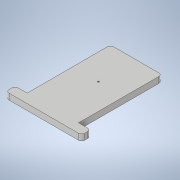
# Autodesk Inventor part: 00_Slider_Mask_Darkfield
Saved by Autodesk Inventor 2022.3 (Build 263350000, 350)
## iProperties
Created: 2021-10-22
Part Number: 00_Slider_Mask_Darkfield
Material: Generic
Document SubType Name: Modeling
Designer: diederichbenedict
Density: 1 g/cm^3
Appearance: Default
Author: diederichbenedict
Autodesk Inventor part; units mm, degrees
ref_plane "YZ Plane" through (0, 0, 0) normal (1, 0, 0) x (0, 1, 0)
ref_plane "XZ Plane" through (0, 0, 0) normal (0, 1, 0) x (-1, 0, 0)
ref_plane "XY Plane" through (0, 0, 0) normal (0, 0, 1) x (1, 0, 0)
sketch "Sketch1" plane through (0, 0, 0) normal (0, 1, 0) x (-1, 0, 0)
  line L0 (-17, 30.1) -> (17, 30.1)
  line L1 (17, 30.1) -> (17, 25)
  line L2 (17, -25) -> (-17, -25)
  line L3 (-17, -25) -> (-17, 25)
  line L4 (9, -19.575) -> (9, 19.575)
  line L5 (9, 19.575) -> (-9, 19.575)
  line L6 (-9, 19.575) -> (-9, -19.575)
  line L7 (-9, -19.575) -> (9, -19.575)
  line L8 (-25, 36.1) -> (25, 36.1)
  line L9 (25, 36.1) -> (25, 30.1)
  line L10 (25, 30.1) -> (-25, 30.1)
  line L11 (-25, 30.1) -> (-25, 36.1)
  line L12 (-25, 36.1) -> (25, 30.1) construction
  line L13 (25, 36.1) -> (-25, 30.1) construction
  line L14 (17, 25) -> (-17, 25)
  line L15 (-17, 25) -> (-17, 30.1)
  line L16 (17, 25) -> (17, -25)
  point P0 (0, 0)
  point P1 (0, 33.1)
  point P2 (0, 30.1)
  point P3 (0, 0)
  point P4 (-17, 0)
  point P5 (-9, 0)
  dimension "d0" = 34
  dimension "d1" = 55.1
  dimension "d2" = 8
  dimension "d3" = 50
  dimension "d4" = 6
  dimension "d18" = 5.1
  dimension "d19" = 50
  dimension "d20" = 25
  constraints: 34 end point, 9 parallel, 6 midpoint, 6 perpendicular, 2 horizontal, 2 horizontal alignment
  measures "d0" distance of L2.start L2.end
  measures "d1" distance of L0.end L2.start
  measures "d2" distance between parallel lines of L1 L4
  measures "d3" distance of L9.end L10.end
  measures "d4" distance of L8.end L9.end
  measures "d18" distance between parallel lines of L14 L0
  measures "d19" distance between parallel lines of L2 L14
  measures "d20" distance from line of L14 point (0, 0)
extrude "Extrusion1" add sketch "Sketch1" along normal blind 4 contours L10 L11 L8 L9 L0 | L0 L1 L14 L15 | L14 L16 L2 L3 | L7 L6 L5 L4
sketch "Sketch2" plane through (0, 4, 0) normal (0, 1, 0) x (1, 0, 0)
  line L0 (25, -30.1) -> (17, -30.1) projected
  line L1 (-25, -30.1) -> (-25, -36.1) projected
  line L2 (-25, -36.1) -> (25, -36.1) projected
  line L3 (25, -36.1) -> (25, -30.1) projected
  line L4 (13.5, 17) -> (-13.5, 17)
  line L5 (-13.5, 17) -> (-13.5, -17)
  line L6 (-13.5, -17) -> (13.5, -17)
  line L7 (13.5, -17) -> (13.5, 17)
  line L8 (13.5, 17) -> (-13.5, -17) construction
  line L9 (-13.5, 17) -> (13.5, -17) construction
  circle A0 centre (0, 0) radius 13.5 construction
  circle A1 centre (0, 0) radius 0.5
  line L10 (-0.4, 0.3) -> (-13.9997, 0.3) construction
  line L11 (-13.9997, 0.3) -> (-13.9997, -0.3) construction
  line L12 (-13.9997, -0.3) -> (-0.4, -0.3) construction
  line L13 (-0.4, -0.3) -> (-0.4, 0.3) construction
  line L14 (0.4, 0.3) -> (13.9718, 0.3) construction
  line L15 (13.9718, 0.3) -> (13.9718, -0.3) construction
  line L16 (13.9718, -0.3) -> (0.4, -0.3) construction
  line L17 (0.4, -0.3) -> (0.4, 0.3) construction
  line L18 (17, -30.1) -> (17, 25) projected
  line L19 (17, 25) -> (-17, 25) projected
  line L20 (-17, 25) -> (-17, -30.1) projected
  line L21 (-17, -30.1) -> (-25, -30.1) projected
  point P0 (13.4967, -0.3)
  point P1 (13.5, -0.3)
  point P2 (13.5, 0)
  point P3 (13.5, 0.3)
  point P4 (13.4967, 0.3)
  point P5 (0.4, -0.3)
  point P6 (0.4, -0.3)
  point P7 (-0.4, -0.3)
  point P8 (-0.4, -0.3)
  point P9 (-13.4967, -0.3)
  point P10 (-13.5, -0.3)
  point P11 (-13.5, 0)
  point P12 (-13.4967, 0.3)
  point P13 (-13.5, 0.3)
  point P14 (-17, 0)
  dimension "d7" = 27
  dimension "d8" = 34
  dimension "d14" = 0.3
  dimension "d15" = 0.3
  dimension "d16" = 1
  constraints: 28 end point, 6 parallel, 3 horizontal, 3 midpoint, 3 perpendicular, 2 centre point, 2 coincident, 2 point on circle, 2 point on line, 1 horizontal alignment
  measures "d7" distance of L6.end L5.end
  measures "d8" distance of L5.end L4.end
  measures "d14" distance from line of point (0, 0) L10
  measures "d15" distance from line of point (0, 0) L12
  measures "d16" diameter of A1
extrude "Extrusion2" cut sketch "Sketch2" against normal through all draft 45 contours A1
sketch "Sketch3" plane through (0, 4, 0) normal (0, 1, 0) x (1, 0, 0)
  line L0 (-13.1847, -19.2539) -> (12.0411, -19.2539) construction
  line L1 (12.0411, -19.2539) -> (12.0411, -24.441) construction
  line L2 (12.0411, -24.441) -> (-13.1847, -24.441) construction
  line L3 (-13.1847, -24.441) -> (-13.1847, -19.2539) construction
  point P0 (0, 0)
  constraints: 2 other
extrude "Extrusion3" [suppressed]
fillet "Fillet1" radius 2 6 edges at (25, 2, 36.1) (25, 2, 30.1) (-25, 2, 36.1) (-25, 2, 30.1) (-17, 2, -25) (17, 2, -25)
sketch "Sketch4" plane through (0, 0, 0) normal (0, -1, 0) x (1, 0, 0)
  line L0 (-15.3446, -7.6834) -> (10.8174, -7.6834) construction
  line L1 (10.8174, -7.6834) -> (10.8174, -21.8309) construction
  line L2 (10.8174, -21.8309) -> (-15.3446, -21.8309) construction
  line L3 (-15.3446, -21.8309) -> (-15.3446, -7.6834) construction
  line L4 (-6.685, -13.4285) -> (-8.6364, -13.4285)
  line L5 (-8.6364, -13.4285) -> (-8.6364, -13.0201)
  line L6 (-8.6364, -13.0201) -> (-7.9103, -13.0201)
  line L7 (-7.9103, -13.0201) -> (-7.9103, -10.3394)
  line L8 (-7.9103, -10.3394) -> (-8.6364, -10.3394)
  line L9 (-8.6364, -10.3394) -> (-8.6364, -9.9731)
  spline S0 degree 2 poles (-8.6364, -9.9731) (-8.2247, -9.9731) (-7.8357, -9.7397) (-7.8098, -9.4156) knots 0 0 0 1 2 2 2
  line L10 (-7.8098, -9.4156) -> (-7.3949, -9.4156)
  line L11 (-7.3949, -9.4156) -> (-7.3949, -13.0201)
  line L12 (-7.3949, -13.0201) -> (-6.685, -13.0201)
  line L13 (-6.685, -13.0201) -> (-6.685, -13.4285)
  line L14 (-0.7531, -13.4285) -> (-0.7531, -11.6911)
  spline S1 degree 2 poles (-0.7531, -11.6911) (-0.7531, -11.4836) (-0.7855, -11.1303) (-0.8373, -11.0331) knots 0 0 0 1 2 2 2
  spline S2 degree 2 poles (-0.8373, -11.0331) (-0.8892, -10.9261) (-1.0869, -10.8224) (-1.2587, -10.8224) knots 0 0 0 1 2 2 2
  spline S3 degree 2 poles (-1.2587, -10.8224) (-1.4143, -10.8224) (-1.7709, -11.0136) (-1.9589, -11.1951) knots 0 0 0 1 2 2 2
  spline S4 degree 2 poles (-1.9589, -11.1951) (-1.9557, -11.2405) (-1.9492, -11.3669) (-1.9492, -11.4512) knots 0 0 0 1 2 2 2
  line L15 (-1.9492, -11.4512) -> (-1.9492, -13.4285)
  line L16 (-1.9492, -13.4285) -> (-2.4549, -13.4285)
  line L17 (-2.4549, -13.4285) -> (-2.4549, -11.6911)
  spline S5 degree 2 poles (-2.4549, -11.6911) (-2.4549, -11.4836) (-2.4873, -11.1303) (-2.5391, -11.0331) knots 0 0 0 1 2 2 2
  spline S6 degree 2 poles (-2.5391, -11.0331) (-2.591, -10.9261) (-2.7887, -10.8224) (-2.9605, -10.8224) knots 0 0 0 1 2 2 2
  spline S7 degree 2 poles (-2.9605, -10.8224) (-3.1226, -10.8224) (-3.4824, -11.0266) (-3.651, -11.1854) knots 0 0 0 1 2 2 2
  line L18 (-3.651, -11.1854) -> (-3.651, -13.4285)
  line L19 (-3.651, -13.4285) -> (-4.1566, -13.4285)
  line L20 (-4.1566, -13.4285) -> (-4.1566, -10.4269)
  line L21 (-4.1566, -10.4269) -> (-3.651, -10.4269)
  line L22 (-3.651, -10.4269) -> (-3.651, -10.7575)
  spline S8 degree 2 poles (-3.651, -10.7575) (-3.4532, -10.5598) (-3.0643, -10.3426) (-2.8309, -10.3426) knots 0 0 0 1 2 2 2
  spline S9 degree 2 poles (-2.8309, -10.3426) (-2.5651, -10.3426) (-2.1534, -10.5857) (-2.0464, -10.8613) knots 0 0 0 1 2 2 2
  spline S10 degree 2 poles (-2.0464, -10.8613) (-1.8163, -10.6052) (-1.3819, -10.3426) (-1.1291, -10.3426) knots 0 0 0 1 2 2 2
  spline S11 degree 2 poles (-1.1291, -10.3426) (-0.9346, -10.3426) (-0.6169, -10.4626) (-0.5002, -10.5987) knots 0 0 0 1 2 2 2
  spline S12 degree 2 poles (-0.5002, -10.5987) (-0.3803, -10.7348) (-0.2474, -11.1433) (-0.2474, -11.4512) knots 0 0 0 1 2 2 2
  line L23 (-0.2474, -11.4512) -> (-0.2474, -13.4285)
  line L24 (-0.2474, -13.4285) -> (-0.7531, -13.4285)
  line L25 (3.8661, -13.4285) -> (3.8661, -11.6911)
  spline S13 degree 2 poles (3.8661, -11.6911) (3.8661, -11.4836) (3.8336, -11.1303) (3.7818, -11.0331) knots 0 0 0 1 2 2 2
  spline S14 degree 2 poles (3.7818, -11.0331) (3.7299, -10.9261) (3.5322, -10.8224) (3.3604, -10.8224) knots 0 0 0 1 2 2 2
  spline S15 degree 2 poles (3.3604, -10.8224) (3.2048, -10.8224) (2.8482, -11.0136) (2.6602, -11.1951) knots 0 0 0 1 2 2 2
  spline S16 degree 2 poles (2.6602, -11.1951) (2.6635, -11.2405) (2.6699, -11.3669) (2.6699, -11.4512) knots 0 0 0 1 2 2 2
  line L26 (2.6699, -11.4512) -> (2.6699, -13.4285)
  line L27 (2.6699, -13.4285) -> (2.1643, -13.4285)
  line L28 (2.1643, -13.4285) -> (2.1643, -11.6911)
  spline S17 degree 2 poles (2.1643, -11.6911) (2.1643, -11.4836) (2.1319, -11.1303) (2.08, -11.0331) knots 0 0 0 1 2 2 2
  spline S18 degree 2 poles (2.08, -11.0331) (2.0281, -10.9261) (1.8304, -10.8224) (1.6586, -10.8224) knots 0 0 0 1 2 2 2
  spline S19 degree 2 poles (1.6586, -10.8224) (1.4965, -10.8224) (1.1367, -11.0266) (0.9682, -11.1854) knots 0 0 0 1 2 2 2
  line L29 (0.9682, -11.1854) -> (0.9682, -13.4285)
  line L30 (0.9682, -13.4285) -> (0.4625, -13.4285)
  line L31 (0.4625, -13.4285) -> (0.4625, -10.4269)
  line L32 (0.4625, -10.4269) -> (0.9682, -10.4269)
  line L33 (0.9682, -10.4269) -> (0.9682, -10.7575)
  spline S20 degree 2 poles (0.9682, -10.7575) (1.1659, -10.5598) (1.5549, -10.3426) (1.7883, -10.3426) knots 0 0 0 1 2 2 2
  spline S21 degree 2 poles (1.7883, -10.3426) (2.0541, -10.3426) (2.4657, -10.5857) (2.5727, -10.8613) knots 0 0 0 1 2 2 2
  spline S22 degree 2 poles (2.5727, -10.8613) (2.8028, -10.6052) (3.2372, -10.3426) (3.49, -10.3426) knots 0 0 0 1 2 2 2
  spline S23 degree 2 poles (3.49, -10.3426) (3.6845, -10.3426) (4.0022, -10.4626) (4.1189, -10.5987) knots 0 0 0 1 2 2 2
  spline S24 degree 2 poles (4.1189, -10.5987) (4.2388, -10.7348) (4.3717, -11.1433) (4.3717, -11.4512) knots 0 0 0 1 2 2 2
  line L34 (4.3717, -11.4512) -> (4.3717, -13.4285)
  line L35 (4.3717, -13.4285) -> (3.8661, -13.4285)
  spline S25 degree 2 poles (-8.1113, -17.2202) (-8.1113, -17.4796) (-8.296, -17.9463) (-8.4613, -18.1084) knots 0 0 0 1 2 2 2
  spline S26 degree 2 poles (-8.4613, -18.1084) (-8.6688, -18.3126) (-9.2296, -18.5233) (-9.6574, -18.5233) knots 0 0 0 1 2 2 2
  line L36 (-9.6574, -18.5233) -> (-10.108, -18.5233)
  line L37 (-10.108, -18.5233) -> (-10.108, -20.0144)
  line L38 (-10.108, -20.0144) -> (-10.6396, -20.0144)
  line L39 (-10.6396, -20.0144) -> (-10.6396, -16.0144)
  line L40 (-10.6396, -16.0144) -> (-9.6348, -16.0144)
  spline S27 degree 2 poles (-9.6348, -16.0144) (-9.2782, -16.0144) (-8.779, -16.1311) (-8.5878, -16.264) knots 0 0 0 1 2 2 2
  spline S28 degree 2 poles (-8.5878, -16.264) (-8.3641, -16.4164) (-8.1113, -16.8864) (-8.1113, -17.2202) knots 0 0 0 1 2 2 2
  spline S29 degree 2 poles (-8.6655, -17.2365) (-8.6655, -17.029) (-8.8082, -16.7243) (-8.954, -16.6271) knots 0 0 0 1 2 2 2
  spline S30 degree 2 poles (-8.954, -16.6271) (-9.0805, -16.5428) (-9.4176, -16.4747) (-9.6672, -16.4747) knots 0 0 0 1 2 2 2
  line L41 (-9.6672, -16.4747) -> (-10.108, -16.4747)
  line L42 (-10.108, -16.4747) -> (-10.108, -18.0695)
  line L43 (-10.108, -18.0695) -> (-9.745, -18.0695)
  spline S31 degree 2 poles (-9.745, -18.0695) (-9.4208, -18.0695) (-9.0221, -17.9658) (-8.8925, -17.8296) knots 0 0 0 1 2 2 2
  spline S32 degree 2 poles (-8.8925, -17.8296) (-8.7725, -17.7097) (-8.6655, -17.4277) (-8.6655, -17.2365) knots 0 0 0 1 2 2 2
  line L44 (-7.1291, -20.0144) -> (-7.6348, -20.0144)
  line L45 (-7.6348, -20.0144) -> (-7.6348, -17.0128)
  line L46 (-7.6348, -17.0128) -> (-7.1291, -17.0128)
  line L47 (-7.1291, -17.0128) -> (-7.1291, -20.0144)
  line L48 (-7.0934, -16.5136) -> (-7.6672, -16.5136)
  line L49 (-7.6672, -16.5136) -> (-7.6672, -15.9885)
  line L50 (-7.6672, -15.9885) -> (-7.0934, -15.9885)
  line L51 (-7.0934, -15.9885) -> (-7.0934, -16.5136)
  line L52 (-4.0302, -20.0144) -> (-4.5359, -20.0144)
  line L53 (-4.5359, -20.0144) -> (-4.5359, -18.3029)
  spline S33 degree 2 poles (-4.5359, -18.3029) (-4.5359, -18.0954) (-4.5748, -17.7389) (-4.6331, -17.6319) knots 0 0 0 1 2 2 2
  spline S34 degree 2 poles (-4.6331, -17.6319) (-4.6947, -17.5185) (-4.9151, -17.4083) (-5.1031, -17.4083) knots 0 0 0 1 2 2 2
  spline S35 degree 2 poles (-5.1031, -17.4083) (-5.2912, -17.4083) (-5.6899, -17.6092) (-5.8811, -17.7713) knots 0 0 0 1 2 2 2
  line L54 (-5.8811, -17.7713) -> (-5.8811, -20.0144)
  line L55 (-5.8811, -20.0144) -> (-6.3868, -20.0144)
  line L56 (-6.3868, -20.0144) -> (-6.3868, -17.0128)
  line L57 (-6.3868, -17.0128) -> (-5.8811, -17.0128)
  line L58 (-5.8811, -17.0128) -> (-5.8811, -17.3467)
  spline S36 degree 2 poles (-5.8811, -17.3467) (-5.6542, -17.1425) (-5.2166, -16.9285) (-4.9702, -16.9285) knots 0 0 0 1 2 2 2
  spline S37 degree 2 poles (-4.9702, -16.9285) (-4.5294, -16.9285) (-4.0302, -17.512) (-4.0302, -18.0663) knots 0 0 0 1 2 2 2
  line L59 (-4.0302, -18.0663) -> (-4.0302, -20.0144)
  line L60 (-0.9638, -20.0144) -> (-1.4694, -20.0144)
  line L61 (-1.4694, -20.0144) -> (-1.4694, -18.3029)
  spline S38 degree 2 poles (-1.4694, -18.3029) (-1.4694, -18.0954) (-1.5083, -17.7389) (-1.5667, -17.6319) knots 0 0 0 1 2 2 2
  spline S39 degree 2 poles (-1.5667, -17.6319) (-1.6283, -17.5185) (-1.8487, -17.4083) (-2.0367, -17.4083) knots 0 0 0 1 2 2 2
  spline S40 degree 2 poles (-2.0367, -17.4083) (-2.2247, -17.4083) (-2.6234, -17.6092) (-2.8147, -17.7713) knots 0 0 0 1 2 2 2
  line L62 (-2.8147, -17.7713) -> (-2.8147, -20.0144)
  line L63 (-2.8147, -20.0144) -> (-3.3203, -20.0144)
  line L64 (-3.3203, -20.0144) -> (-3.3203, -15.8361)
  line L65 (-3.3203, -15.8361) -> (-2.8147, -15.8361)
  line L66 (-2.8147, -15.8361) -> (-2.8147, -17.3467)
  spline S41 degree 2 poles (-2.8147, -17.3467) (-2.5878, -17.1425) (-2.1501, -16.9285) (-1.9038, -16.9285) knots 0 0 0 1 2 2 2
  spline S42 degree 2 poles (-1.9038, -16.9285) (-1.463, -16.9285) (-0.9638, -17.512) (-0.9638, -18.0663) knots 0 0 0 1 2 2 2
  line L67 (-0.9638, -18.0663) -> (-0.9638, -20.0144)
  spline S43 degree 2 poles (2.2129, -18.5136) (2.2129, -19.2721) (1.4836, -20.0987) (0.8742, -20.0987) knots 0 0 0 1 2 2 2
  spline S44 degree 2 poles (0.8742, -20.0987) (0.2486, -20.0987) (-0.4678, -19.2462) (-0.4678, -18.5136) knots 0 0 0 1 2 2 2
  spline S45 degree 2 poles (-0.4678, -18.5136) (-0.4678, -17.7616) (0.2712, -16.9285) (0.8742, -16.9285) knots 0 0 0 1 2 2 2
  spline S46 degree 2 poles (0.8742, -16.9285) (1.4836, -16.9285) (2.2129, -17.7583) (2.2129, -18.5136) knots 0 0 0 1 2 2 2
  spline S47 degree 2 poles (1.691, -18.5136) (1.691, -17.9301) (1.2664, -17.3629) (0.8742, -17.3629) knots 0 0 0 1 2 2 2
  spline S48 degree 2 poles (0.8742, -17.3629) (0.4819, -17.3629) (0.0541, -17.9301) (0.0541, -18.5136) knots 0 0 0 1 2 2 2
  spline S49 degree 2 poles (0.0541, -18.5136) (0.0541, -19.0809) (0.4819, -19.6643) (0.8742, -19.6643) knots 0 0 0 1 2 2 2
  spline S50 degree 2 poles (0.8742, -19.6643) (1.2631, -19.6643) (1.691, -19.0906) (1.691, -18.5136) knots 0 0 0 1 2 2 2
  line L68 (3.2469, -20.0144) -> (2.7413, -20.0144)
  line L69 (2.7413, -20.0144) -> (2.7413, -15.8361)
  line L70 (2.7413, -15.8361) -> (3.2469, -15.8361)
  line L71 (3.2469, -15.8361) -> (3.2469, -20.0144)
  spline S51 degree 2 poles (5.2923, -20.0825) (4.5727, -20.0825) (3.7818, -19.2754) (3.7818, -18.5298) knots 0 0 0 1 2 2 2
  spline S52 degree 2 poles (3.7818, -18.5298) (3.7818, -17.7972) (4.55, -16.9285) (5.1691, -16.9285) knots 0 0 0 1 2 2 2
  spline S53 degree 2 poles (5.1691, -16.9285) (5.4479, -16.9285) (5.879, -17.0906) (6.0379, -17.2624) knots 0 0 0 1 2 2 2
  spline S54 degree 2 poles (6.0379, -17.2624) (6.1999, -17.4342) (6.3717, -17.9301) (6.3717, -18.2899) knots 0 0 0 1 2 2 2
  line L72 (6.3717, -18.2899) -> (6.3717, -18.5655)
  line L73 (6.3717, -18.5655) -> (4.2939, -18.5655)
  spline S55 degree 2 poles (4.2939, -18.5655) (4.2939, -19.0873) (4.8191, -19.6416) (5.2858, -19.6416) knots 0 0 0 1 2 2 2
  spline S56 degree 2 poles (5.2858, -19.6416) (5.4511, -19.6416) (5.7721, -19.5671) (5.9017, -19.5087) knots 0 0 0 1 2 2 2
  spline S57 degree 2 poles (5.9017, -19.5087) (6.0379, -19.4439) (6.2259, -19.3305) (6.2875, -19.2786) knots 0 0 0 1 2 2 2
  line L74 (6.2875, -19.2786) -> (6.3166, -19.2786)
  line L75 (6.3166, -19.2786) -> (6.3166, -19.8296)
  spline S58 degree 2 poles (6.3166, -19.8296) (6.2291, -19.8653) (5.9633, -19.969) (5.8596, -19.9982) knots 0 0 0 1 2 2 2
  spline S59 degree 2 poles (5.8596, -19.9982) (5.7137, -20.0403) (5.4738, -20.0825) (5.2923, -20.0825) knots 0 0 0 1 2 2 2
  spline S60 degree 2 poles (5.879, -18.1797) (5.8725, -17.9755) (5.7883, -17.6773) (5.7072, -17.5768) knots 0 0 0 1 2 2 2
  spline S61 degree 2 poles (5.7072, -17.5768) (5.6197, -17.4634) (5.3442, -17.3434) (5.14, -17.3434) knots 0 0 0 1 2 2 2
  spline S62 degree 2 poles (5.14, -17.3434) (4.939, -17.3434) (4.657, -17.4634) (4.5403, -17.5801) knots 0 0 0 1 2 2 2
  spline S63 degree 2 poles (4.5403, -17.5801) (4.4268, -17.7) (4.3101, -17.9885) (4.2939, -18.1797) knots 0 0 0 1 2 2 2
  line L76 (4.2939, -18.1797) -> (5.879, -18.1797)
  point P0 (0, 0)
  constraints: 2 other
extrude "Extrusion4" cut sketch "Sketch4" against normal blind 2
sketch "Sketch5" plane through (0, 0, 0) normal (0, -1, 0) x (1, 0, 0)
  circle A0 centre (0, 0) radius 4.5 projected
  circle A1 centre (0, 0) radius 0.5 projected
  circle A2 centre (0, 0) radius 10
  circle A3 centre (0, 0) radius 9.5
  dimension "d23" = 20
  dimension "d24" = 19
  constraints: 2 centre point, 2 coincident
  measures "d23" diameter of A2
  measures "d24" diameter of A3
extrude "Extrusion5" [suppressed]
sketch "Sketch6" plane through (0, 0, 0) normal (0, -1, 0) x (1, 0, 0)
  line L0 (17, 30.1) -> (16.3, 30.1)
  line L1 (15.5, 30.1) -> (15.5, 29.5)
  line L2 (15.5, -25) -> (17, -25)
  line L3 (17, -25) -> (17, 30.1)
  line L4 (15.5, -0.5) -> (11.5, -0.5)
  line L5 (11.5, -0.5) -> (11.5, 0.5)
  line L6 (11.5, 0.5) -> (15.5, 0.5)
  line L7 (15.5, 0.5) -> (15.5, -0.5)
  line L8 (15.5, -24.5) -> (15.5, -25)
  line L9 (15.5, -15.5) -> (11.5, -15.5)
  line L10 (11.5, -15.5) -> (11.5, -14.5)
  line L11 (11.5, -14.5) -> (15.5, -14.5)
  line L12 (15.5, -14.5) -> (15.5, -15.5)
  line L13 (15.5, 25.5) -> (11.5, 25.5)
  line L14 (11.5, 25.5) -> (11.5, 24.5)
  line L15 (11.5, 24.5) -> (15.5, 24.5)
  line L16 (15.5, 24.5) -> (15.5, 25.5)
  line L17 (15.5, 20.5) -> (11.5, 20.5)
  line L18 (11.5, 20.5) -> (11.5, 19.5)
  line L19 (11.5, 19.5) -> (15.5, 19.5)
  line L20 (15.5, 19.5) -> (15.5, 20.5)
  line L21 (15.5, 15.5) -> (11.5, 15.5)
  line L22 (11.5, 15.5) -> (11.5, 14.5)
  line L23 (11.5, 14.5) -> (15.5, 14.5)
  line L24 (15.5, 14.5) -> (15.5, 15.5)
  line L25 (15.5, 10.5) -> (11.5, 10.5)
  line L26 (11.5, 10.5) -> (11.5, 9.5)
  line L27 (11.5, 9.5) -> (15.5, 9.5)
  line L28 (15.5, 9.5) -> (15.5, 10.5)
  line L29 (15.5, -4.5) -> (11.5, -4.5)
  line L30 (11.5, -4.5) -> (11.5, -5.5)
  line L31 (11.5, -5.5) -> (15.5, -5.5)
  line L32 (15.5, -5.5) -> (15.5, -4.5)
  line L33 (15.5, -9.5) -> (11.5, -9.5)
  line L34 (11.5, -9.5) -> (11.5, -10.5)
  line L35 (11.5, -10.5) -> (15.5, -10.5)
  line L36 (15.5, -10.5) -> (15.5, -9.5)
  line L37 (15.5, 5.5) -> (11.5, 5.5)
  line L38 (11.5, 4.5) -> (15.5, 4.5)
  line L39 (15.5, 4.5) -> (15.5, 5.5)
  line L40 (11.5, 5.5) -> (11.5, 4.5)
  line L41 (15.5, -19.5) -> (11.5, -19.5)
  line L42 (11.5, -20.5) -> (15.5, -20.5)
  line L43 (15.5, -20.5) -> (15.5, -19.5)
  line L44 (11.5, -19.5) -> (11.5, -20.5)
  line L45 (16.3, 30.1) -> (16.3, -25)
  arc A0 (15, -25) -> (17, -23) centre (15, -23) ccw projected
  line L46 (15.5, 30.5) -> (11.5, 30.5)
  line L47 (11.5, 30.5) -> (11.5, 29.5)
  line L48 (11.5, 29.5) -> (15.5, 29.5)
  line L49 (15.5, 29.5) -> (15.5, 30.1)
  line L50 (15.5, 30.5) -> (16.3, 30.5)
  line L51 (17, 30.5) -> (17, 30.1)
  line L52 (16.3, 30.5) -> (16.3, 30.1)
  line L53 (16.3, 30.1) -> (15.5, 30.1)
  line L54 (16.3, 30.1) -> (16.3, 30.0559)
  line L55 (16.3, 30.5) -> (17, 30.5)
  line L56 (15.5, 29.5) -> (15.5, -25)
  line L57 (15.5, 30.1) -> (15.5, 30.5)
  point P0 (0, 0)
  point P1 (13.5, 24.5)
  point P2 (13.5, 25.5)
  point P3 (13.5, 0.5)
  point P4 (11.5, 0)
  point P5 (11.5, 25)
  point P6 (11.5, 20)
  point P7 (11.5, -15)
  point P8 (11.5, 15)
  point P9 (11.5, 10)
  point P10 (11.5, -5)
  point P11 (11.5, -10)
  point P12 (11.5, 5)
  point P13 (11.5, -20)
  point P14 (13.5, -0.5)
  point P15 (15.5, 24.75)
  point P16 (15.5, 19.75)
  point P17 (15.5, 15.25)
  point P18 (15.5, 14.75)
  point P19 (15.5, 10.25)
  point P20 (15.5, 9.75)
  point P21 (15.5, 5.25)
  point P22 (15.5, 4.75)
  point P23 (15.5, 0.25)
  point P24 (15.5, -4.75)
  point P25 (15.5, -5.25)
  point P26 (15.5, -9.75)
  point P27 (15.5, -10.25)
  point P28 (15.5, -14.75)
  point P29 (15.5, -19.75)
  point P30 (15.5, -20.25)
  point P31 (15.5, -24.9365)
  point P32 (16.3, -24.5199)
  point P33 (11.5, 30)
  point P34 (15.5, 19.5)
  point P35 (15.5, 15.5)
  point P36 (15.5, 14.5)
  point P37 (15.5, 10.5)
  point P38 (15.5, 9.5)
  point P39 (15.5, 5.5)
  point P40 (15.5, 4.5)
  point P41 (15.5, 0.5)
  point P42 (15.5, -4.5)
  point P43 (15.5, -5.5)
  point P44 (15.5, -9.5)
  point P45 (15.5, -10.5)
  point P46 (15.5, -14.5)
  point P47 (15.5, -19.5)
  point P48 (15.5, -20.5)
  point P49 (15.5, -24.9365)
  dimension "d27" = 55.1
  dimension "d28" = 1.5
  dimension "d30" = 1
  dimension "d31" = 1
  dimension "d33" = 1
  dimension "d38" = 1
  dimension "d40" = 1
  dimension "d42" = 1
  dimension "d44" = 1
  dimension "d51" = 1
  dimension "d55" = 1
  dimension "d62" = 5
  dimension "d63" = 5
  dimension "d64" = 5
  dimension "d65" = 5
  dimension "d66" = 5
  dimension "d67" = 4
  dimension "d68" = 5
  dimension "d69" = 5
  dimension "d70" = 5
  dimension "d71" = 5
  dimension "d72" = 0.7
  dimension "d73" = 1
  dimension "d78" = 5
  dimension "d79" = 1
  dimension "d80" = 4
  dimension "d81" = 4
  constraints: 112 end point, 25 parallel, 19 horizontal, 15 midpoint, 13 perpendicular, 10 vertical alignment, 4 point on line, 3 vertical, 1 horizontal alignment, 14 other
  measures "d27" distance of L2.end L0.start
  measures "d30" distance of point (13.5, 24.5) point (13.5, 25.5)
  measures "d31" distance between parallel lines of L19 L17
  measures "d33" distance between parallel lines of L9 L11
  measures "d38" distance between parallel lines of L23 L21
  measures "d40" distance between parallel lines of L27 L25
  measures "d42" distance between parallel lines of L31 L29
  measures "d44" distance between parallel lines of L35 L33
  measures "d51" distance between parallel lines of L38 L37
  measures "d55" distance between parallel lines of L42 L41
  measures "d62" distance of point (11.5, 0) point (11.5, 5)
  measures "d63" distance of point (11.5, 10) point (11.5, 5)
  measures "d64" distance of point (11.5, 15) point (11.5, 10)
  measures "d65" distance of point (11.5, 20) point (11.5, 15)
  measures "d66" distance of point (11.5, 25) point (11.5, 20)
  measures "d67" distance of L13.start L13.end
  measures "d68" distance of point (11.5, -5) point (11.5, 0)
  measures "d69" distance of point (11.5, -10) point (11.5, -5)
  measures "d70" distance of point (11.5, -15) point (11.5, -10)
  measures "d71" distance of point (11.5, -20) point (11.5, -15)
  measures "d72" distance between parallel lines of L45 L3
  measures "d73" distance from line of point (13.5, -0.5) L6
  measures "d78" distance of point (11.5, 25) point (11.5, 30)
  measures "d79" distance between parallel lines of L46 L48
  measures "d80" distance of L46.start L46.end
  measures "d81" distance of L17.start L17.end
extrude "Extrusion6" cut sketch "Sketch6" against normal blind 1 contours L53 L57 L50 L52 | L45 A0 L8 L56 L43 L12 L36 L32 L7 L39 L28 L24 L20 L16 L1 L53 | L1 L48 L47 L46 L57 | L16 L15 L14 L13 | L42 L44 L41 L43 | L20 L19 L18 L17 | L9 L10 L11 L12 | L24 L23 L22 L21 | L35 L34 L33 L36 | L28 L27 L26 L25 | L31 L30 L29 L32 | L39 L38 L40 L37 | L4 L5 L6 L7
equation "\"d30\" = d73"
equation "\"d31\" = d73"
equation "\"d33\" = d73"
equation "\"d38\" = d73"
equation "\"d40\" = d73"
equation "\"d42\" = d73"
equation "\"d44\" = d73"
equation "\"d51\" = d73"
equation "\"d55\" = d73"
equation "\"d63\" = d62"
equation "\"d64\" = d62"
equation "\"d65\" = d62"
equation "\"d66\" = d62"
equation "\"d68\" = d62"
equation "\"d69\" = d68"
equation "\"d70\" = d69"
equation "\"d71\" = d62"
equation "\"d79\" = d30"
equation "\"d81\" = d67"
body "Solid1"
